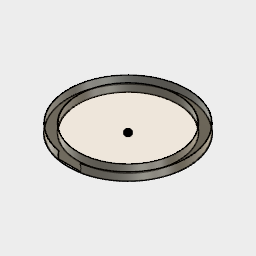
Jenkins_Monitor_Outer_Ring_Cover v1 (Autodesk Fusion 360 design; units mm, degrees)
Autodesk Fusion 360 part; units mm, degrees
sketch "Sketch1" plane through (0, 0, 0) normal (0, 0, 1) x (1, 0, 0)
  circle A0 centre (0, 0) radius 69.3
  circle A1 centre (0, 0) radius 81.7
  circle A2 centre (0, 0) radius 68.3
  circle A3 centre (0, 0) radius 82.7
  dimension "d1" = 138.6
  dimension "d2" = 163.4
  dimension "d3" = 136.6
  dimension "d4" = 165.4
  measures "d1" diameter of A0
  measures "d2" diameter of A1
  measures "d3" diameter of A2
  measures "d4" diameter of A3
extrude "Extrude1" add sketch "Sketch1" along normal blind 1 contours A0 | A1 | A3
extrude "Extrude2" add sketch "Sketch1" along normal blind 11
ref_plane "WorkPlane1" through (0, -82.7, 0) normal (0, 1, 0) x (0, 0, 1)
sketch "Sketch2" plane through (0, -82.7, 0) normal (0, 1, 0) x (1, 0, 0)
  circle A0 centre (0, -5) radius 16
  dimension "d10" = 32
  measures "d10" diameter of A0
extrude "Extrude3" cut sketch "Sketch2" along normal blind 2.5
equation "d3 = d1 - 2 mm"
equation "d4 = d2 + 2 mm"
equation "d9 = -1 * ( d4 / 2 )"
